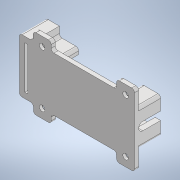
# Autodesk Inventor part: SyringeCasing
Saved by Autodesk Inventor 2022 (Build 260153000, 153)
## iProperties
Created: 2022-06-05
Part Number: SyringeCasing
Material: Generic
Document SubType Name: Modeling
Designer: frede
Density: 1 g/cm^3
Appearance: Default
Author: frede
Autodesk Inventor part; units mm, degrees
ref_plane "YZ Plane" through (0, 0, 0) normal (1, 0, 0) x (0, 1, 0)
ref_plane "XZ Plane" through (0, 0, 0) normal (0, 1, 0) x (-1, 0, 0)
ref_plane "XY Plane" through (0, 0, 0) normal (0, 0, 1) x (1, 0, 0)
sketch "Sketch1" plane through (0, 0, 0) normal (0, 0, 1) x (1, 0, 0)
  line L0 (-33.557, 36.1315) -> (-43.657, 36.1315)
  line L1 (-43.657, 36.1315) -> (-43.657, -3.0685)
  line L2 (-43.657, -3.0685) -> (-33.457, -3.0685)
  line L3 (40.043, 3.5815) -> (40.043, 29.4815)
  line L4 (35.943, 25.1065) -> (35.943, 7.9565) construction
  line L5 (35.943, 7.9565) -> (-29.957, 7.9565) construction
  line L6 (35.943, 25.1065) -> (-29.957, 25.1065) construction
  line L7 (-37.557, 25.3815) -> (-29.957, 25.3815) construction
  line L8 (-29.957, 7.6815) -> (-29.957, 25.3815) construction
  line L9 (-37.557, 7.6815) -> (-29.957, 7.6815) construction
  line L10 (-37.557, 1.0315) -> (-37.557, 6.1295) construction
  line L11 (-39.557, 1.0315) -> (-37.557, 1.0315) construction
  line L12 (-39.557, 6.1295) -> (-39.557, 1.0315) construction
  line L13 (-39.557, 13.2232) -> (-39.557, 6.1295) construction
  line L14 (-39.557, 19.8398) -> (-39.557, 13.2232) construction
  line L15 (-39.557, 26.9336) -> (-39.557, 19.8398) construction
  line L16 (-39.557, 32.0315) -> (-39.557, 26.9336) construction
  line L17 (-39.557, 32.0315) -> (-37.557, 32.0315) construction
  line L18 (-37.557, 26.9336) -> (-37.557, 32.0315) construction
  line L19 (-37.557, 19.8398) -> (-37.557, 26.9336) construction
  line L20 (-37.557, 6.1295) -> (-37.557, 13.2232) construction
  line L21 (-33.557, 36.1315) -> (-33.557, 29.4815) construction
  line L22 (-33.557, 29.4815) -> (40.043, 29.4815) construction
  line L23 (35.943, 25.1065) -> (-29.957, 25.1065) construction
  line L24 (-29.957, 25.3815) -> (-29.957, 25.1065) construction
  line L25 (-29.957, 25.3815) -> (-37.557, 25.3815) construction
  line L26 (-37.557, 25.3815) -> (-37.557, 32.0315) construction
  line L27 (-37.557, 32.0315) -> (-39.557, 32.0315) construction
  line L28 (-39.557, 32.0315) -> (-39.557, 1.0315) construction
  line L29 (-39.557, 1.0315) -> (-37.557, 1.0315) construction
  line L30 (-37.557, 1.0315) -> (-37.557, 7.6815) construction
  line L31 (-37.557, 7.6815) -> (-29.957, 7.6815) construction
  line L32 (-29.957, 7.6815) -> (-29.957, 7.9565) construction
  line L33 (-29.957, 7.9565) -> (35.943, 7.9565) construction
  line L34 (35.943, 7.9565) -> (35.943, 25.1065) construction
  line L35 (-29.857, 7.8565) -> (36.043, 7.8565)
  line L36 (36.043, 7.8565) -> (36.043, 25.2065)
  line L37 (36.043, 25.2065) -> (-29.857, 25.2065)
  line L38 (-29.857, 25.2065) -> (-29.857, 25.4815)
  line L39 (-29.857, 25.4815) -> (-37.457, 25.4815)
  line L40 (-37.457, 25.4815) -> (-37.457, 32.1315)
  line L41 (-37.457, 32.1315) -> (-39.657, 32.1315)
  line L42 (-39.657, 32.1315) -> (-39.657, 0.9315)
  line L43 (-39.657, 0.9315) -> (-37.457, 0.9315)
  line L44 (-37.457, 0.9315) -> (-37.457, 7.5815)
  line L45 (-37.457, 7.5815) -> (-29.857, 7.5815)
  line L46 (-29.857, 7.5815) -> (-29.857, 7.8565)
  line L47 (-33.557, 36.1315) -> (-33.557, 29.4815)
  line L48 (-33.557, 29.4815) -> (40.043, 29.4815)
  line L49 (-33.457, -3.0685) -> (-33.457, 3.5815)
  line L50 (-33.457, 3.5815) -> (40.043, 3.5815)
  line L51 (-33.457, 36.1315) -> (-33.557, 36.1315)
  line L52 (-33.457, 36.1315) -> (-33.557, 36.1315)
  point P0 (0, 0)
  dimension "d6" = 0.1
  dimension "d7" = 4
  dimension "d8" = 4
  dimension "d9" = 4
  dimension "d10" = 4
  dimension "d11" = 4
  dimension "d12" = 4
  dimension "d13" = 4
  dimension "d14" = 4
  constraints: 84 end point, 15 perpendicular, 9 horizontal, 5 collinear, 4 parallel, 1 point on line, 18 other
  measures "d6" distance between parallel lines of L5 L35
  measures "d7" distance between parallel lines of L45 L50
  measures "d8" distance between parallel lines of L44 L49
  measures "d9" distance between parallel lines of L43 L2
  measures "d10" distance between parallel lines of L42 L1
  measures "d11" distance between parallel lines of L41 L0
  measures "d12" distance between parallel lines of L26 L21
  measures "d13" distance between parallel lines of L39 L22
  measures "d14" distance between parallel lines of L36 L3
extrude "Extrusion1" add sketch "Sketch1" along normal blind 16
sketch "Sketch2" plane through (0, 0, 16) normal (0, 0, 1) x (1, 0, 0)
  line L0 (-43.657, 36.1315) -> (-43.657, -3.0685) projected
  line L1 (-43.657, -3.0685) -> (-43.657, 36.1315)
  line L2 (40.043, 36.1315) -> (40.043, -3.0685)
  line L3 (-43.657, -3.0685) -> (-33.457, -3.0685) projected
  line L4 (40.043, 3.5815) -> (40.043, 29.4815) projected
  line L5 (40.043, 29.4815) -> (27.043, 29.4815) construction
  line L6 (27.043, 36.1315) -> (27.043, 42.4815)
  line L7 (27.043, 42.4815) -> (40.043, 42.4815)
  line L8 (40.043, 42.4815) -> (40.043, 29.4815)
  line L9 (-33.557, 29.4815) -> (-33.557, 36.1315) construction
  line L10 (-33.557, 29.4815) -> (-20.557, 29.4815) construction
  line L11 (-20.557, 36.1315) -> (-20.557, 42.4815)
  line L12 (-20.557, 42.4815) -> (-33.557, 42.4815)
  line L13 (-33.557, 42.4815) -> (-33.557, 36.1315)
  line L14 (-33.457, 3.5815) -> (40.043, 3.5815) construction
  line L15 (-20.557, 3.5815) -> (-20.457, 3.5815)
  line L16 (-20.457, -3.0685) -> (-20.457, -9.4185)
  line L17 (-20.457, -9.4185) -> (-33.457, -9.4185)
  line L18 (-33.457, -9.4185) -> (-33.457, -3.0685)
  line L19 (40.043, 3.5815) -> (27.043, 3.5815) construction
  line L20 (27.043, -3.0685) -> (27.043, -9.4185)
  line L21 (27.043, -9.4185) -> (40.043, -9.4185)
  line L22 (40.043, -9.4185) -> (40.043, 3.5815)
  line L23 (27.043, -3.0685) -> (-20.457, -3.0685)
  line L24 (-33.457, -3.0685) -> (-43.657, -3.0685)
  line L25 (-43.657, 36.1315) -> (-33.557, 36.1315)
  line L26 (-20.557, 36.1315) -> (27.043, 36.1315)
  point P0 (0, 0)
  point P1 (-38.557, -3.0685)
  point P2 (40.043, 16.5315)
  dimension "d60" = 13
  dimension "d61" = 13
  dimension "d62" = 13
  dimension "d63" = 13
  dimension "d64" = 13
  dimension "d65" = 13
  dimension "d66" = 13
  dimension "d67" = 13
  constraints: 44 end point, 13 parallel, 6 horizontal, 6 perpendicular, 4 midpoint, 2 point on line
  measures "d60" distance of L6.end L7.end
  measures "d61" distance of L5.end L6.end
  measures "d62" distance of L12.end L11.end
  measures "d63" distance of L11.end L10.end
  measures "d64" distance of L16.end L17.end
  measures "d65" distance of L15.end L16.end
  measures "d66" distance of L21.end L20.end
  measures "d67" distance of L20.end L19.end
extrude "Extrusion2" add sketch "Sketch2" along normal blind 3
sketch "Sketch3" plane through (40.043, 3.5815, 0) normal (1, 0, 0) x (0, 0, -1)
  line L0 (0, 15.95) -> (-16, 15.95)
  line L1 (-16, 15.95) -> (-16, 9.95)
  line L2 (-16, 9.95) -> (0, 9.95)
  line L3 (0, 9.95) -> (0, 15.95)
  line L4 (0, 0) -> (0, 25.9) construction
  line L5 (0, 25.9) -> (-16, 25.9) construction
  line L6 (0, 0) -> (-16, 0) construction
  line L7 (-16, 21.625) -> (-16, 4.275) construction
  point P0 (0, -3.5815)
  point P1 (0, 12.95)
  dimension "d19" = 6
  dimension "d21" = 0
  constraints: 8 end point, 2 midpoint, 2 parallel, 1 horizontal, 1 perpendicular
  measures "d19" distance of L1.end L0.end
  measures "d21" distance between parallel lines of L7 L1
extrude "Extrusion3" cut sketch "Sketch3" against normal blind 4
fillet "Fillet1" radius 3 2 edges at (38.043, 19.5315, 16) (38.043, 13.5315, 16)
sketch "Sketch4" plane through (-43.657, -3.0685, 0) normal (-1, 0, 0) x (0, 0, 1)
  line L0 (0, 27.5) -> (16, 27.5)
  line L1 (16, 27.5) -> (16, 11.7)
  line L2 (16, 11.7) -> (0, 11.7)
  line L3 (0, 11.7) -> (0, 27.5)
  line L4 (0, 39.2) -> (0, 0) construction
  line L5 (0, 39.2) -> (19, 39.2) construction
  line L6 (0, 0) -> (19, 0) construction
  line L7 (19, 39.2) -> (19, 0) construction
  point P0 (0, 3.0685)
  point P1 (0, 19.6)
  dimension "d25" = 15.8
  dimension "d28" = 11.7
  dimension "d29" = 11.7
  dimension "d30" = 3
  constraints: 8 end point, 2 midpoint, 2 parallel, 1 horizontal, 1 perpendicular
  measures "d25" distance of L0.end L1.end
  measures "d28" distance between parallel lines of L0 L5
  measures "d29" distance between parallel lines of L6 L2
  measures "d30" distance between parallel lines of L7 L1
extrude "Extrusion4" cut sketch "Sketch4" against normal blind 4
chamfer "Chamfer1" distance 7.5 angle 45 2 edges at (-41.657, 8.6315, 16) (-41.657, 24.4315, 16)
sketch "Sketch5" plane through (0, 0, 16) normal (0, 0, -1) x (-1, 0, 0)
  circle A0 centre (-33.543, 35.9815) radius 2
  circle A1 centre (27.057, 35.9815) radius 2
  circle A2 centre (27.057, -2.9185) radius 2
  circle A3 centre (-33.543, -2.9185) radius 2
  line L0 (-40.043, 29.4815) -> (-40.043, 3.5815) projected
  line L1 (-40.043, 36.1315) -> (33.557, 36.1315) projected
  line L2 (-40.043, 29.4815) -> (33.557, 29.4815) projected
  line L3 (-40.043, -9.4185) -> (-40.043, 3.5815) projected
  line L4 (33.457, -3.0685) -> (-27.043, -3.0685) projected
  line L5 (33.457, -3.0685) -> (33.457, 3.5815) projected
  line L6 (20.557, 42.4815) -> (33.557, 42.4815) projected
  line L7 (33.457, -9.4185) -> (20.457, -9.4185) projected
  line L8 (-27.043, -9.4185) -> (-40.043, -9.4185) projected
  point P0 (0, 0)
  point P1 (-40.043, -3.0685)
  point P2 (27.057, 42.4815)
  point P3 (-33.543, -9.4185)
  dimension "d39" = 4
  dimension "d68" = 6.5
  dimension "d69" = 6.5
  constraints: 4 centre point, 4 vertical alignment, 3 equal radius, 2 horizontal alignment, 2 midpoint
  measures "d39" diameter of A3
  measures "d68" distance from line of L7 A2.centre
  measures "d69" distance from line of L6 A1.centre
extrude "Extrusion5" cut sketch "Sketch5" against normal blind 4
chamfer "Chamfer2" distance 1 angle 45 4 edges at (35.543, 35.9815, 16) (35.543, -2.9185, 16) (-25.057, 35.9815, 16) (-25.057, -2.9185, 16)
chamfer "Chamfer3" distance 0.275 angle 45 2 edges at (-29.857, 25.2065, 8) (-29.857, 7.8565, 8)
sketch "Sketch6" plane through (0, 0, 0) normal (0, 0, -1) x (-1, 0, 0)
  line L0 (37.457, 0.9315) -> (39.657, 0.9315) projected
  line L1 (39.657, 32.1315) -> (37.457, 32.1315)
  line L2 (37.457, 32.1315) -> (37.457, 0.9315)
  line L3 (37.457, 0.9315) -> (39.657, 0.9315)
  line L4 (39.657, 0.9315) -> (39.657, 32.1315)
  point P0 (0, 0)
  constraints: 8 end point, 2 parallel, 1 horizontal, 1 perpendicular
extrude "Extrusion6" cut sketch "Sketch6" against normal through all
sketch "Sketch7" plane through (-33.557, 29.4815, 0) normal (0, 1, 0) x (1, 0, 0)
  line L0 (3.7, 0) -> (3.7, -16) construction
  line L1 (3.975, -16) -> (3.975, 0) construction
  line L2 (69.6, 0) -> (69.6, -16) construction
  line L3 (13.975, 0) -> (59.6, 0)
  line L4 (59.6, 0) -> (59.6, -16)
  line L5 (59.6, -16) -> (13.975, -16)
  line L6 (13.975, -16) -> (13.975, 0)
  line L7 (73.6, -16) -> (0, -16) construction
  point P0 (33.557, 0)
  point P1 (36.7875, -16)
  point P2 (36.8, -16)
  dimension "d56" = 10
  dimension "d57" = 10
  constraints: 8 end point, 2 midpoint, 2 parallel, 1 horizontal, 1 horizontal alignment, 1 perpendicular, 1 point on line
  measures "d56" distance between parallel lines of L6 L1
  measures "d57" distance between parallel lines of L4 L2
extrude "Extrusion7" cut sketch "Sketch7" against normal through all
fillet "Fillet2" radius 2 24 edges at (-33.557, 42.4815, 17.5) (-20.557, 42.4815, 17.5) (27.043, 42.4815, 17.5) (40.043, 42.4815, 17.5) (27.043, -9.4185, 17.5) (40.043, -9.4185, 17.5) (-20.457, -9.4185, 17.5) (-33.457, -9.4185, 17.5) (-43.657, -3.0685, 9.5) (-43.657, 36.1315, 9.5) (-19.582, 29.4815, 8) (-19.582, 3.5815, 8) (40.043, 29.4815, 8) (40.043, 3.5815, 8) (26.043, 3.5815, 8) (26.043, 29.4815, 8) (27.043, 36.1315, 17.5) (-20.557, 36.1315, 17.5) (-33.557, 36.1315, 17.5) (-33.557, 29.4815, 8) (-33.457, 3.5815, 8) (-20.457, -3.0685, 17.5) (27.043, -3.0685, 17.5) (-33.457, -3.0685, 17.5)
equation "\"d28\" = d29"
equation "\"d69\" = d68"
body "Solid1"
